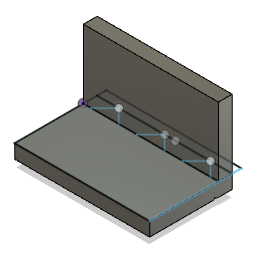
hot stake test v4 (Autodesk Fusion 360 design; units mm, degrees)
Autodesk Fusion 360 part; units mm, degrees
sketch "5mm layout" plane through (0, 0, 0) normal (0, 1, 0) x (1, 0, 0)
  line L0 (0, 0) -> (30, 0)
  line L1 (30, 0) -> (30, 20)
  line L2 (30, 20) -> (0, 20)
  line L3 (0, 20) -> (0, 0)
  line L4 (0, 15) -> (30, 15) construction
  circle A0 centre (5, 15) radius 2.5
  circle A1 centre (15, 15) radius 2.5
  circle A2 centre (25, 15) radius 2.5
  line L5 (0, 10) -> (30, 10)
  dimension "d1" = 30
  dimension "d2" = 20
  dimension "d3" = 5
  dimension "d4" = 5
  dimension "d5" = 5
  dimension "d6" = 5
  dimension "d7" = 5
  dimension "d8" = 5
  constraint horizontal L0
  constraint vertical L1
  constraint horizontal L2
  constraint vertical L3
  constraint coincident L0.start L3.end
  constraint coincident L3 L4.start
  constraint coincident L1 L4.end
  constraint perpendicular L1 L4
  constraint coincident L4 A0.centre
  constraint midpoint L4 A1.centre
  constraint coincident L4 A2.centre
  constraint midpoint L3 L5.start
  constraint midpoint L1 L5.end
  measures "d1" distance of L0.start L0.end
  measures "d2" distance of L0.start L2.end
  measures "d3" diameter of A0
  measures "d4" diameter of A1
  measures "d5" diameter of A2
  measures "d6" distance of L2 L4
  measures "d7" distance of L4.start A0.centre
  measures "d8" distance of L1 A2.centre
extrude "Extrude1" add sketch "5mm layout" against normal blind 5 makes body 1
extrude "Extrude2" add sketch "5mm layout" along normal blind 20 separate body contours L1 L2 L3 L5 | A0 | A1 | A2 makes body 2
extrude "Extrude3" add sketch "5mm layout" against normal blind 6 contours A0 | A1 | A2 bodies 2
chamfer "Chamfer1" distance 1 angle 45 3 edges at (22.6692, -5, -14.096) (12.6692, -5, -14.096) (2.6692, -5, -14.096) on bodies 1
move_face "OffsetFaces1" offset -0.2 3 faces at (7.4969, -2.6667, -14.8754) (17.4969, -2.6667, -14.8754) (27.4969, -2.6667, -14.8754) on bodies 1
sketch "5mm rebates" plane through (0, -6, 0) normal (0, -1, 0) x (1, 0, 0)
  circle A0 centre (25, -15) radius 2.5
  circle A1 centre (25, -15) radius 1.5
  circle A2 centre (14.984, -15.0131) radius 1.5
  circle A3 centre (4.9839, -15.0131) radius 1.5
  dimension "d17" = 3
  dimension "d18" = 3
  dimension "d19" = 3
  constraint concentric A0 A1
  measures "d17" diameter of A1
  measures "d18" diameter of A2
  measures "d19" diameter of A3
extrude "Extrude4" cut sketch "5mm rebates" against normal blind 1 contours A1 | A2 | A3 bodies 2
sketch "2m layout" plane through (0, 0, 0) normal (0, 1, 0) x (1, 0, 0)
  circle A0 centre (0, 0) radius 1
  circle A1 centre (5, 0) radius 1
  circle A2 centre (10, 0) radius 1
  line L0 (-3, -1.5) -> (13, -1.5)
  line L1 (13, -1.5) -> (13, 1.5)
  line L2 (13, 1.5) -> (-3, 1.5)
  line L3 (-3, 1.5) -> (-3, -1.5)
  line L4 (13, -1.5) -> (-3, -1.5)
  line L5 (-3, -1.5) -> (-3, -16.5)
  line L6 (-3, -16.5) -> (13, -16.5)
  line L7 (13, -16.5) -> (13, -1.5)
  dimension "d22" = 2
  dimension "d25" = 5
  dimension "d26" = 0
  dimension "d27" = 3
  dimension "d28" = 3
  dimension "d29" = 3
  dimension "d30" = 1.5
  dimension "d31" = 15
  constraint coincident A0.centre origin
  constraint horizontal L0
  constraint vertical L1
  constraint horizontal L2
  constraint vertical L3
  constraint horizontal L4
  constraint vertical L5
  constraint horizontal L6
  constraint vertical L7
  measures "d22" diameter of A0
  measures "d27" distance of L0.start L2.end
  measures "d28" distance of A0.centre L3
  measures "d29" distance of A2.centre L1
  measures "d30" distance of A1.centre L2
  measures "d31" distance of L0.end L6.end
extrude "Extrude5" add sketch "2m layout" along normal blind 3 separate body makes body 3
extrude "Extrude6" add sketch "2m layout" against normal blind 15 separate body contours A0 | A1 | A2 | L0 L1 L2 L3 L4 makes body 4
extrude "Extrude7" add sketch "2m layout" along normal blind 4 contours A0 | A1 | A2 bodies 4
chamfer "Chamfer2" distance 0.7 angle 45 3 edges at (-0.9323, 3, -0.3616) (4.0677, 3, -0.3616) (9.0677, 3, -0.3616) on bodies 3
sketch "3mm dovetail" plane through (0, 0, 0) normal (0, 1, 0) x (1, 0, 0)
  line L0 (0, 0) -> (29.4548, 0)
  line L1 (29.4548, 3) -> (0, 3)
  line L2 (0, 3) -> (0, 0)
  line L3 (14.7274, 0) -> (14.7274, 3) construction
  line L4 (14.7274, 3) -> (17.7274, 0)
  line L5 (14.7274, 3) -> (17.0507, 3) construction
  line L6 (14.7274, 3) -> (11.7274, 0)
  line L7 (4.7274, 3) -> (1.7274, 0)
  line L8 (4.7274, 3) -> (7.7274, 0)
  line L9 (24.7274, 3) -> (21.7274, 0)
  line L10 (24.7274, 3) -> (27.7274, 0)
  line L11 (29.4548, 3) -> (29.4548, 0)
  line L12 (0, 0) -> (29.4548, 0)
  line L13 (29.4548, 0) -> (29.4548, -15)
  line L14 (29.4548, -15) -> (0, -15)
  line L15 (0, -15) -> (0, 0)
  line L16 (0, 3) -> (29.4548, 3)
  line L17 (29.4548, 3) -> (29.4548, 5)
  line L18 (29.4548, 5) -> (0, 5)
  line L19 (0, 5) -> (0, 3)
  dimension "d40" = 3
  dimension "d41" = 45
  dimension "d46" = 15
  dimension "d54" = 2
  constraint horizontal L0
  constraint horizontal L1
  constraint vertical L2
  constraint coincident L0.start L2.end
  constraint midpoint L0 L3.start
  constraint midpoint L1 L3.end
  constraint horizontal L5
  constraint symmetric L4.start L3 L5.start
  constraint coincident L0 L7.end
  constraint coincident L0 L8.end
  constraint coincident L0 L6.end
  constraint coincident L0 L4.end
  constraint coincident L0 L10.end
  constraint coincident L0 L9.end
  constraint perpendicular L0 L11
  constraint horizontal L12
  constraint vertical L13
  constraint horizontal L14
  constraint vertical L15
  constraint horizontal L16
  constraint vertical L17
  constraint horizontal L18
  constraint vertical L19
  measures "d40" distance of L0.start L1.end
  measures "d41" angle of L4 L5
  measures "d46" distance of L0.start L14.end
  measures "d54" distance of L1.end L18.end
extrude "Extrude8" add sketch "3mm dovetail" against normal blind 3 separate body contours L0 L1 L2 L7 L12 L16 | L0 L12 L13 L14 L15 | L1 L16 L17 L18 L19 | L0 L1 L6 L8 L12 L16 | L0 L1 L4 L9 L12 L16 | L0 L1 L10 L11 L12 L16 makes body 5
extrude "Extrude9" add sketch "3mm dovetail" against normal blind 4.5 separate body contours L0 L7 L8 L12 | L0 L4 L6 L12 | L0 L9 L10 L12 makes body 6 at (3.7274, -1.5, 0) makes body 7 at (13.7274, -1.5, 0) makes body 8 at (23.7274, -1.5, 0)
extrude "Extrude10" add sketch "3mm dovetail" along normal blind 15 contours L0 L1 L2 L7 L12 L16 | L0 L7 L8 L12 | L0 L1 L6 L8 L12 L16 | L0 L4 L6 L12 | L0 L1 L4 L9 L12 L16 | L0 L1 L10 L11 L12 L16 | L0 L9 L10 L12 bodies 6 7 8
move_face "OffsetFaces2" offset -0.1 6 faces at (25.7274, -1.5, -2) (23.7274, -1.5, -2) (16.7274, -3, -1) (13.7274, -1.5, -2) (6.7274, -3, -1) (3.7274, -1.5, -2) on bodies 6
chamfer "Chamfer3" distance 1 angle 45 9 edges at (26.2274, -3, -1.5) (23.2274, -3, -1.5) (24.7274, -3, 0) (16.2274, -3, -1.5) (14.7274, -3, 0) (13.2274, -3, -1.5) (6.2274, -3, -1.5) (4.7274, -3, 0) (3.2274, -3, -1.5) on bodies 5
extrude "Extrude11" cut sketch "3mm dovetail" against normal blind 3 contours L1 L16 L17 L18 L19 bodies 5
hidden bodies 1 2 3 4
named bodies: "5mm holes", "5mmm pins", "2mm holes", "2mm pins", "3mm dovetail holes", "3mm dovetail pins"
